Autodesk Fusion 360 part; units mm, degrees
(part 2 of 2)
  line L143 (-32.4194, -45.1753, 132.2927) -> (-24.3664, -49.1663, 133.2373) construction
  line L144 (-24.3664, -49.1663, 133.2373) -> (-16.3142, -53.1569, 134.1819) construction
  line L145 (-16.3142, -53.1569, 134.1819) -> (-7.27, -55.1267, 135.1265) construction
  line L146 (-7.27, -55.1267, 135.1265) -> (1.7125, -54.8463, 136.071) construction
  line L147 (1.7125, -54.8463, 136.071) -> (10.6942, -54.5658, 137.0155) construction
  line L148 (10.6942, -54.5658, 137.0155) -> (19.597, -52.0361, 137.96) construction
  line L149 (19.597, -52.0361, 137.96) -> (27.3842, -47.5516, 138.9044) construction
  line L150 (27.3842, -47.5516, 138.9044) -> (35.1706, -43.0675, 139.8488) construction
  line L151 (35.1706, -43.0675, 139.8488) -> (41.8265, -36.6377, 140.7932) construction
  line L152 (41.8265, -36.6377, 140.7932) -> (46.577, -29.0109, 141.7376) construction
  line L153 (46.577, -29.0109, 141.7376) -> (51.327, -21.3848, 142.6819) construction
  line L154 (51.327, -21.3848, 142.6819) -> (54.1627, -12.5764, 143.6262) construction
  line L155 (54.1627, -12.5764, 143.6262) -> (54.754, -3.6114, 144.5705) construction
  line L156 (54.754, -3.6114, 144.5705) -> (55.3453, 5.3528, 145.5148) construction
  line L157 (55.3453, 5.3528, 145.5148) -> (53.6914, 14.4564, 146.459) construction
  line L158 (53.6914, 14.4564, 146.459) -> (49.9848, 22.6398, 147.4032) construction
  line L159 (49.9848, 22.6398, 147.4032) -> (46.2786, 30.8225, 148.3474) construction
  line L160 (46.2786, 30.8225, 148.3474) -> (40.5272, 38.0694, 149.2915) construction
  line L161 (40.5272, 38.0694, 149.2915) -> (33.4001, 43.5371, 150.2356) construction
  line L162 (33.4001, 43.5371, 150.2356) -> (26.2735, 49.0044, 151.1797) construction
  line L163 (26.2735, 49.0044, 151.1797) -> (17.7851, 52.6822, 152.1238) construction
  line L164 (17.7851, 52.6822, 152.1238) -> (8.9225, 54.1427, 153.0678) construction
  line L165 (8.9225, 54.1427, 153.0678) -> (0.0607, 55.6031, 154.0118) construction
  line L166 (0.0607, 55.6031, 154.0118) -> (-9.1583, 54.8438, 154.9558) construction
  line L167 (-9.1583, 54.8438, 154.9558) -> (-17.6617, 51.953, 155.8998) construction
  line L168 (-17.6617, 51.953, 155.8998) -> (-26.1644, 49.0624, 156.8437) construction
  line L169 (-26.1644, 49.0624, 156.8437) -> (-33.9354, 44.0464, 157.7876) construction
  line L170 (-33.9354, 44.0464, 157.7876) -> (-40.0708, 37.4884, 158.7315) construction
  line L171 (-40.0708, 37.4884, 158.7315) -> (-46.2057, 30.9309, 159.6753) construction
  line L172 (-46.2057, 30.9309, 159.6753) -> (-50.6934, 22.8442, 160.6191) construction
  line L173 (-50.6934, 22.8442, 160.6191) -> (-53.0121, 14.1689, 161.5629) construction
  line L174 (-53.0121, 14.1689, 161.5629) -> (-55.3307, 5.4944, 162.5067) construction
  line L175 (-55.3307, 5.4944, 162.5067) -> (-55.476, -3.7522, 163.4504) construction
  line L176 (-55.476, -3.7522, 163.4504) -> (-53.4314, -12.4953, 164.3941) construction
  line L177 (-53.4314, -12.4953, 164.3941) -> (-51.3869, -21.2378, 165.3378) construction
  line L178 (-51.3869, -21.2378, 165.3378) -> (-47.1566, -29.4603, 166.2815) construction
  line L179 (-47.1566, -29.4603, 166.2815) -> (-41.2325, -36.2067, 167.2251) construction
  line L180 (-41.2325, -36.2067, 167.2251) -> (-35.3088, -42.9527, 168.1687) construction
  line L181 (-35.3088, -42.9527, 168.1687) -> (-27.7029, -48.2099, 169.1123) construction
  line L182 (-27.7029, -48.2099, 169.1123) -> (-19.2988, -51.3673, 170.0559) construction
  line L183 (-19.2988, -51.3673, 170.0559) -> (-10.8954, -54.5245, 170.9994) construction
  line L184 (-10.8954, -54.5245, 170.9994) -> (-1.7102, -55.5761, 171.9429) construction
  line L185 (-1.7102, -55.5761, 171.9429) -> (7.1893, -54.4, 172.8864) construction
  line L186 (7.1893, -54.4, 172.8864) -> (16.088, -53.224, 173.8298) construction
  line L187 (16.088, -53.224, 173.8298) -> (24.6841, -49.8228, 174.7733) construction
  line L188 (24.6841, -49.8228, 174.7733) -> (31.9784, -44.5918, 175.7167) construction
  line L189 (31.9784, -44.5918, 175.7167) -> (39.2722, -39.3611, 176.6601) construction
  line L190 (39.2722, -39.3611, 176.6601) -> (45.2505, -32.3109, 177.6034) construction
  line L191 (45.2505, -32.3109, 177.6034) -> (49.2187, -24.2604, 178.5468) construction
  line L192 (49.2187, -24.2604, 178.5468) -> (53.1866, -16.2104, 179.4901) construction
  line L193 (53.1866, -16.2104, 179.4901) -> (55.1371, -7.1757, 180.4333) construction
  line L194 (55.1371, -7.1757, 180.4333) -> (54.8437, 1.7942, 181.3766) construction
  line L195 (54.8437, 1.7942, 181.3766) -> (54.5502, 10.7635, 182.3198) construction
  line L196 (54.5502, 10.7635, 182.3198) -> (52.0137, 19.6507, 183.263) construction
  line L197 (52.0137, 19.6507, 183.263) -> (47.5288, 27.4237, 184.2062) construction
  line L198 (47.5288, 27.4237, 184.2062) -> (43.0443, 35.196, 185.1494) construction
  line L199 (43.0443, 35.196, 185.1494) -> (36.6202, 41.8393, 186.0925) construction
  line L200 (36.6202, 41.8393, 186.0925) -> (29.0026, 46.5821, 187.0356) construction
  line L201 (29.0026, 46.5821, 187.0356) -> (21.3857, 51.3245, 187.9787) construction
  line L202 (21.3857, 51.3245, 187.9787) -> (12.5901, 54.1576, 188.9218) construction
  line L203 (12.5901, 54.1576, 188.9218) -> (3.6372, 54.7523, 189.8648) construction
  line L204 (3.6372, 54.7523, 189.8648) -> (-5.315, 55.347, 190.8078) construction
  line L205 (-5.315, 55.347, 190.8078) -> (-14.4074, 53.7026, 191.7508) construction
  line L206 (-14.4074, 53.7026, 191.7508) -> (-22.5842, 50.01, 192.6938) construction
  line L207 (-22.5842, 50.01, 192.6938) -> (-30.7604, 46.3177, 193.6367) construction
  line L208 (-30.7604, 46.3177, 193.6367) -> (-38.0056, 40.5845, 194.5796) construction
  line L209 (-38.0056, 40.5845, 194.5796) -> (-43.4787, 33.4761, 195.5226) construction
  line L210 (-43.4787, 33.4761, 195.5226) -> (-48.9513, 26.3682, 196.4654) construction
  line L211 (-48.9513, 26.3682, 196.4654) -> (-52.6417, 17.8989, 197.4083) construction
  line L212 (-52.6417, 17.8989, 197.4083) -> (-54.1214, 9.0512, 198.3511) construction
  line L213 (-54.1214, 9.0512, 198.3511) -> (-55.6009, 0.2041, 199.2939) construction
  line L214 (-55.6009, 0.2041, 199.2939) -> (-54.8673, -9.0044, 200.2367) construction
  line L215 (-54.8673, -9.0044, 200.2367) -> (-52.0057, -17.5057, 201.1795) construction
  line L216 (-52.0057, -17.5057, 201.1795) -> (-49.1443, -26.0063, 202.1222) construction
  line L217 (-49.1443, -26.0063, 202.1222) -> (-44.1607, -33.7835, 203.0649) construction
  line L218 (-44.1607, -33.7835, 203.0649) -> (-37.6331, -39.9349, 204.0076) construction
  line L219 (-37.6331, -39.9349, 204.0076) -> (-31.106, -46.0858, 204.9502) construction
  line L220 (-31.106, -46.0858, 204.9502) -> (-23.0477, -50.5993, 205.8929) construction
  line L221 (-23.0477, -50.5993, 205.8929) -> (-14.3931, -52.9517, 206.8355) construction
  line L222 (-14.3931, -52.9517, 206.8355) -> (-5.7391, -55.304, 207.7781) construction
  line L223 (-5.7391, -55.304, 207.7781) -> (3.4946, -55.4911, 208.7207) construction
  line L224 (3.4946, -55.4911, 208.7207) -> (12.2368, -53.4912, 209.6632) construction
  line L225 (12.2368, -53.4912, 209.6632) -> (20.9783, -51.4915, 210.6058) construction
  line L226 (20.9783, -51.4915, 210.6058) -> (29.2118, -47.3089, 211.5483) construction
  line L227 (29.2118, -47.3089, 211.5483) -> (35.9821, -41.4287, 212.4908) construction
  line L228 (35.9821, -41.4287, 212.4908) -> (42.7519, -35.5489, 213.4332) construction
  line L229 (42.7519, -35.5489, 213.4332) -> (48.0459, -27.9829, 214.3757) construction
  line L230 (48.0459, -27.9829, 214.3757) -> (51.25, -19.6082, 215.3181) construction
  line L231 (51.25, -19.6082, 215.3181) -> (54.4539, -11.2341, 216.2605) construction
  line L232 (54.4539, -11.2341, 216.2605) -> (55.5622, -2.0673, 217.2029) construction
  line L233 (55.5622, -2.0673, 217.2029) -> (54.4464, 6.8291, 218.1452) construction
  line L234 (54.4464, 6.8291, 218.1452) -> (53.3306, 15.7249, 219.0875) construction
  line L235 (53.3306, 15.7249, 219.0875) -> (49.9931, 24.3334, 220.0299) construction
  line L236 (49.9931, 24.3334, 220.0299) -> (44.8209, 31.6565, 220.9722) construction
  line L237 (44.8209, 31.6565, 220.9722) -> (39.649, 38.9791, 221.9144) construction
  line L238 (39.649, 38.9791, 221.9144) -> (32.6524, 45.0026, 222.8567) construction
  line L239 (32.6524, 45.0026, 222.8567) -> (24.6424, 49.0285, 223.7989) construction
  line L240 (24.6424, 49.0285, 223.7989) -> (16.6329, 53.0542, 224.7411) construction
  line L241 (16.6329, 53.0542, 224.7411) -> (7.6252, 55.075, 225.6833) construction
  line L242 (7.6252, 55.075, 225.6833) -> (-1.3364, 54.8567, 226.6255) construction
  line L243 (-1.3364, 54.8567, 226.6255) -> (-10.2974, 54.6384, 227.5676) construction
  line L244 (-10.2974, 54.6384, 227.5676) -> (-19.1954, 52.1817, 228.5097) construction
  line L245 (-19.1954, 52.1817, 228.5097) -> (-26.999, 47.7713, 229.4518) construction
  line L246 (-26.999, 47.7713, 229.4518) -> (-34.8021, 43.3612, 230.3939) construction
  line L247 (-34.8021, 43.3612, 230.3939) -> (-41.4962, 37.0061, 231.336) construction
  line L248 (-41.4962, 37.0061, 231.336) -> (-46.3054, 29.4425, 232.278) construction
  line L249 (-46.3054, 29.4425, 232.278) -> (-51.1143, 21.8793, 233.22) construction
  line L250 (-51.1143, 21.8793, 233.22) -> (-54.0294, 13.1222, 234.162) construction
  line L251 (-54.0294, 13.1222, 234.162) -> (-54.7131, 4.1858, 235.104) construction
  line L252 (-54.7131, 4.1858, 235.104) -> (-55.3967, -4.7501, 236.046) construction
  line L253 (-55.3967, -4.7501, 236.046) -> (-53.8479, -13.8482, 236.9879) construction
  line L254 (-53.8479, -13.8482, 236.9879) -> (-50.2459, -22.0544, 237.9298) construction
  line L255 (-50.2459, -22.0544, 237.9298) -> (-46.6442, -30.2601, 238.8717) construction
  line L256 (-46.6442, -30.2601, 238.8717) -> (-40.9965, -37.5585, 239.8136) construction
  line L257 (-40.9965, -37.5585, 239.8136) -> (-33.9571, -43.1041, 240.7555) construction
  line L258 (-33.9571, -43.1041, 240.7555) -> (-26.9181, -48.6493, 241.6973) construction
  line L259 (-26.9181, -48.6493, 241.6973) -> (-18.501, -52.4314, 242.6391) construction
  line L260 (-18.501, -52.4314, 242.6391) -> (-9.6808, -54.0123, 243.581) construction
  line L261 (-9.6808, -54.0123, 243.581) -> (-0.8611, -55.5931, 244.5227) construction
  line L262 (-0.8611, -55.5931, 244.5227) -> (8.345, -54.9699, 245.4645) construction
  line L263 (8.345, -54.9699, 245.4645) -> (16.8713, -52.215, 246.4062) construction
  line L264 (16.8713, -52.215, 246.4062) -> (25.397, -49.4602, 247.3479) construction
  line L265 (25.397, -49.4602, 247.3479) -> (33.2267, -44.5792, 248.2897) construction
  line L266 (33.2267, -44.5792, 248.2897) -> (39.4538, -38.1372, 249.2314) construction
  line L267 (39.4538, -38.1372, 249.2314) -> (45.6805, -31.6955, 250.173) construction
  line L268 (45.6805, -31.6955, 250.173) -> (50.2929, -23.7052, 251.1147) construction
  line L269 (50.2929, -23.7052, 251.1147) -> (52.7569, -15.0915, 252.0563) construction
  line L270 (52.7569, -15.0915, 252.0563) -> (55.2208, -6.4784, 252.9979) construction
  line L271 (55.2208, -6.4784, 252.9979) -> (55.5318, 2.7418, 253.9395) construction
  line L272 (55.5318, 2.7418, 253.9395) -> (53.6541, 11.5014, 254.8811) construction
  line L273 (53.6541, 11.5014, 254.8811) -> (51.7765, 20.2606, 255.8226) construction
  line L274 (51.7765, 20.2606, 255.8226) -> (47.7139, 28.5426, 256.7642) construction
  line L275 (47.7139, 28.5426, 256.7642) -> (41.9366, 35.3888, 257.7057) construction
  line L276 (41.9366, 35.3888, 257.7057) -> (36.1596, 42.2347, 258.6472) construction
  line L277 (36.1596, 42.2347, 258.6472) -> (28.6791, 47.6318, 259.5887) construction
  line L278 (28.6791, 47.6318, 259.5887) -> (20.361, 50.9556, 260.5301) construction
  line L279 (20.361, 50.9556, 260.5301) -> (12.0434, 54.2792, 261.4716) construction
  line L280 (12.0434, 54.2792, 261.4716) -> (2.904, 55.5233, 262.413) construction
  line L281 (2.904, 55.5233, 262.413) -> (-5.9994, 54.5441, 263.3544) construction
  line L282 (-5.9994, 54.5441, 263.3544) -> (-14.9023, 53.5648, 264.2958) construction
  line L283 (-14.9023, 53.5648, 264.2958) -> (-23.5523, 50.3642, 265.2372) construction
  line L284 (-23.5523, 50.3642, 265.2372) -> (-30.9484, 45.3127, 266.1785) construction
  line L285 (-30.9484, 45.3127, 266.1785) -> (-38.3441, 40.2615, 267.1199) construction
  line L286 (-38.3441, 40.2615, 267.1199) -> (-44.472, 33.3691, 268.0612) construction
  line L287 (-44.472, 33.3691, 268.0612) -> (-48.6231, 25.4331, 269.0025) construction
  line L288 (-48.6231, 25.4331, 269.0025) -> (-52.7739, 17.4976, 269.9438) construction
  line L289 (-52.7739, 17.4976, 269.9438) -> (-54.9402, 8.5336, 270.8851) construction
  line L290 (-54.9402, 8.5336, 270.8851) -> (-54.8714, -0.4217, 271.8263) construction
  line L291 (-54.8714, -0.4217, 271.8263) -> (-54.8026, -9.3765, 272.7675) construction
  line L292 (-54.8026, -9.3765, 272.7675) -> (-52.499, -18.3057, 273.7088) construction
  line L293 (-52.499, -18.3057, 273.7088) -> (-48.2271, -26.1762, 274.65) construction
  line L294 (-48.2271, -26.1762, 274.65) -> (-43.9555, -34.0463, 275.5911) construction
  line L295 (-43.9555, -34.0463, 275.5911) -> (-37.7238, -40.8429, 276.5323) construction
  line L296 (-37.7238, -40.8429, 276.5323) -> (-30.2531, -45.7798, 277.4735) construction
  line L297 (-30.2531, -45.7798, 277.4735) -> (-22.7828, -50.7165, 278.4146) construction
  line L298 (-22.7828, -50.7165, 278.4146) -> (-14.0877, -53.7844, 279.3557) construction
  line L299 (-14.0877, -53.7844, 279.3557) -> (-5.1734, -54.6286, 280.2968) construction
  line L300 (-5.1734, -54.6286, 280.2968) -> (3.7404, -55.4727, 281.2379) construction
  line L301 (3.7404, -55.4727, 281.2379) -> (12.8563, -54.0919, 282.179) construction
  line L302 (12.8563, -54.0919, 282.179) -> (21.1202, -50.6457, 283.12) construction
  line L303 (21.1202, -50.6457, 283.12) -> (29.3837, -47.1996, 284.0611) construction
  line L304 (29.3837, -47.1996, 284.0611) -> (36.7795, -41.695, 285.0021) construction
  line L305 (36.7795, -41.695, 285.0021) -> (42.4524, -34.7684, 285.9431) construction
  line L306 (42.4524, -34.7684, 285.9431) -> (48.125, -27.8421, 286.8841) construction
  line L307 (48.125, -27.8421, 286.8841) -> (52.0641, -19.5071, 287.8251) construction
  line L308 (52.0641, -19.5071, 287.8251) -> (53.8143, -10.7271, 288.766) construction
  line L309 (53.8143, -10.7271, 288.766) -> (55.5644, -1.9475, 289.707) construction
  line L310 (55.5644, -1.9475, 289.707) -> (55.1224, 7.2604, 290.6479) construction
  line L311 (55.1224, 7.2604, 290.6479) -> (52.5395, 15.832, 291.5888) construction
  line L312 (52.5395, 15.832, 291.5888) -> (49.8436, 24.7785, 292.5709) construction
  line L313 (49.8436, 24.7785, 292.5709) -> (44.8171, 33.0118, 293.553) construction
  line L314 (44.8171, 33.0118, 293.553) -> (38.0914, 39.498, 294.535) construction
  line L315 (38.0914, 39.498, 294.535) -> (31.4707, 45.8829, 295.5018) construction
  line L316 (31.4707, 45.8829, 295.5018) -> (23.2186, 50.5623, 296.4685) construction
  line L317 (23.2186, 50.5623, 296.4685) -> (14.3404, 52.966, 297.4353) construction
  line L318 (14.3404, 52.966, 297.4353) -> (5.6009, 55.3322, 298.3869) construction
  line L319 (5.6009, 55.3322, 298.3869) -> (-3.7272, 55.4899, 299.3385) construction
  line L320 (-3.7272, 55.4899, 299.3385) -> (-12.5417, 53.4205, 300.2901) construction
  line L321 (-12.5417, 53.4205, 300.2901) -> (-21.2944, 51.3656, 301.2351) construction
  line L322 (-21.2944, 51.3656, 301.2351) -> (-29.5237, 47.1193, 302.1801) construction
  line L323 (-29.5237, 47.1193, 302.1801) -> (-36.2702, 41.1766, 303.125) construction
  line L324 (-36.2702, 41.1766, 303.125) -> (-43.0156, 35.2351, 304.0698) construction
  line L325 (-43.0156, 35.2351, 304.0698) -> (-48.2657, 27.6092, 305.0146) construction
  line L326 (-48.2657, 27.6092, 305.0146) -> (-51.4089, 19.1877, 305.9594) construction
  line L327 (-51.4089, 19.1877, 305.9594) -> (-54.5516, 10.7677, 306.904) construction
  line L328 (-54.5516, 10.7677, 306.904) -> (-55.582, 1.5686, 307.8486) construction
  line L329 (-55.582, 1.5686, 307.8486) -> (-54.3801, -7.338, 308.7932) construction
  line L330 (-54.3801, -7.338, 308.7932) -> (-53.1785, -16.243, 309.7376) construction
  line L331 (-53.1785, -16.243, 309.7376) -> (-49.7478, -24.8384, 310.682) construction
  line L332 (-49.7478, -24.8384, 310.682) -> (-44.4874, -32.1234, 311.6265) construction
  line L333 (-44.4874, -32.1234, 311.6265) -> (-39.228, -39.4072, 312.5707) construction
  line L334 (-39.228, -39.4072, 312.5707) -> (-32.1497, -45.3669, 313.515) construction
  line L335 (-32.1497, -45.3669, 313.515) -> (-24.0766, -49.3088, 314.4593) construction
  line L336 (-24.0766, -49.3088, 314.4593) -> (-16.005, -53.2501, 315.4034) construction
  line L337 (-16.005, -53.2501, 315.4034) -> (-6.9543, -55.1667, 316.3475) construction
  line L338 (-6.9543, -55.1667, 316.3475) -> (2.0222, -54.8357, 317.2916) construction
  line L339 (2.0222, -54.8357, 317.2916) -> (10.997, -54.5048, 318.2355) construction
  line L340 (10.997, -54.5048, 318.2355) -> (19.8805, -51.9276, 319.1795) construction
  line L341 (19.8805, -51.9276, 319.1795) -> (27.639, -47.4039, 320.1234) construction
  line L342 (27.639, -47.4039, 320.1234) -> (35.3962, -42.8811, 321.0672) construction
  line L343 (35.3962, -42.8811, 321.0672) -> (42.0141, -36.4211, 322.011) construction
  line L344 (42.0141, -36.4211, 322.011) -> (46.7229, -28.7753, 322.9548) construction
  line L345 (46.7229, -28.7753, 322.9548) -> (51.4309, -21.1308, 323.8984) construction
  line L346 (51.4309, -21.1308, 323.8984) -> (54.2216, -12.3155, 324.842) construction
  line L347 (54.2216, -12.3155, 324.842) -> (54.7704, -3.3543, 325.7856) construction
  line L348 (54.7704, -3.3543, 325.7856) -> (55.3191, 5.6054, 326.7291) construction
  line L349 (55.3191, 5.6054, 326.7291) -> (53.6257, 14.6938, 327.6726) construction
  line L350 (53.6257, 14.6938, 327.6726) -> (49.887, 22.8547, 328.616) construction
  line L351 (49.887, 22.8547, 328.616) -> (46.1488, 31.0143, 329.5594) construction
  line L352 (46.1488, 31.0143, 329.5594) -> (40.3732, 38.2309, 330.5027) construction
  line L353 (40.3732, 38.2309, 330.5027) -> (33.2311, 43.6663, 331.446) construction
  line L354 (33.2311, 43.6663, 331.446) -> (26.0901, 49.1007, 332.3892) construction
  line L355 (26.0901, 49.1007, 332.3892) -> (17.5967, 52.744, 333.3323) construction
  line L356 (17.5967, 52.744, 333.3323) -> (8.7376, 54.1729, 334.2755) construction
  line L357 (8.7376, 54.1729, 334.2755) -> (-0.1203, 55.6016, 335.2185) construction
  line L358 (-0.1203, 55.6016, 335.2185) -> (-9.3269, 54.8138, 336.1616) construction
  line L359 (-9.3269, 54.8138, 336.1616) -> (-17.8133, 51.9012, 337.1046) construction
  line L360 (-17.8133, 51.9012, 337.1046) -> (-26.2984, 48.989, 338.0475) construction
  line L361 (-26.2984, 48.989, 338.0475) -> (-34.0472, 43.958, 338.9904) construction
  line L362 (-34.0472, 43.958, 338.9904) -> (-40.1604, 37.3924, 339.9333) construction
  line L363 (-40.1604, 37.3924, 339.9333) -> (-46.2726, 30.8277, 340.876) construction
  line L364 (-46.2726, 30.8277, 340.876) -> (-50.7379, 22.7413, 341.8188) construction
  line L365 (-50.7379, 22.7413, 341.8188) -> (-53.0381, 14.0716, 342.7615) construction
  line L366 (-53.0381, 14.0716, 342.7615) -> (-55.3379, 5.4032, 343.7041) construction
  line L367 (-55.3379, 5.4032, 343.7041) -> (-55.4689, -3.8318, 344.6467) construction
  line L368 (-55.4689, -3.8318, 344.6467) -> (-53.4158, -12.562, 345.5893) construction
  line L369 (-53.4158, -12.562, 345.5893) -> (-51.3629, -21.2909, 346.5318) construction
  line L370 (-51.3629, -21.2909, 346.5318) -> (-47.1306, -29.4985, 347.4743) construction
  line L371 (-47.1306, -29.4985, 347.4743) -> (-41.2097, -36.2327, 348.4168) construction
  line L372 (-41.2097, -36.2327, 348.4168) -> (-35.2895, -42.9661, 349.3591) construction
  line L373 (-35.2895, -42.9661, 349.3591) -> (-27.6925, -48.2137, 350.3015) construction
  line L374 (-27.6925, -48.2137, 350.3015) -> (-19.2995, -51.3671, 351.2438) construction
  line L375 (-19.2995, -51.3671, 351.2438) -> (-10.9077, -54.52, 352.186) construction
  line L376 (-10.9077, -54.52, 352.186) -> (-1.7361, -55.5733, 353.1282) construction
  line L377 (-1.7361, -55.5733, 353.1282) -> (7.152, -54.4049, 354.0705) construction
  line L378 (7.152, -54.4049, 354.0705) -> (16.039, -53.2366, 355.0125) construction
  line L379 (16.039, -53.2366, 355.0125) -> (24.6256, -49.8494, 355.9546) construction
  line L380 (24.6256, -49.8494, 355.9546) -> (31.9168, -44.6359, 356.8967) construction
  line L381 (31.9168, -44.6359, 356.8967) -> (39.2071, -39.423, 357.8387) construction
  line L382 (39.2071, -39.423, 357.8387) -> (45.1883, -32.3942, 358.7807) construction
  line L383 (45.1883, -32.3942, 358.7807) -> (49.1676, -24.3638, 359.7226) construction
  line L384 (49.1676, -24.3638, 359.7226) -> (53.1464, -16.3344, 360.6645) construction
  line L385 (53.1464, -16.3344, 360.6645) -> (55.1161, -7.319, 361.6064) construction
  line L386 (55.1161, -7.319, 361.6064) -> (54.8485, 1.6381, 362.5482) construction
  line L387 (54.8485, 1.6381, 362.5482) -> (54.5811, 10.5941, 363.4899) construction
  line L388 (54.5811, 10.5941, 363.4899) -> (52.0774, 19.4749, 364.4317) construction
  line L389 (52.0774, 19.4749, 364.4317) -> (47.6276, 27.2518, 365.3734) construction
  line L390 (47.6276, 27.2518, 365.3734) -> (43.1783, 35.0278, 366.315) construction
  line L391 (43.1783, 35.0278, 366.315) -> (36.7917, 41.6855, 367.2566) construction
  line L392 (36.7917, 41.6855, 367.2566) -> (29.2073, 46.454, 368.1983) construction
  line L393 (29.2073, 46.454, 368.1983) -> (21.6238, 51.2221, 369.1398) construction
  line L394 (21.6238, 51.2221, 369.1398) -> (12.8572, 54.0923, 370.0813) construction
  line L395 (12.8572, 54.0923, 370.0813) -> (3.9223, 54.7326, 371.0228) construction
  line L396 (3.9223, 54.7326, 371.0228) -> (-5.0117, 55.3729, 371.9642) construction
  line L397 (-5.0117, 55.3729, 371.9642) -> (-14.0969, 53.7824, 372.9056) construction
  line L398 (-14.0969, 53.7824, 372.9056) -> (-22.2821, 50.1453, 373.847) construction
  line L399 (-22.2821, 50.1453, 373.847) -> (-30.4663, 46.5087, 374.7883) construction
  line L400 (-30.4663, 46.5087, 374.7883) -> (-37.7351, 40.8328, 375.7296) construction
  line L401 (-37.7351, 40.8328, 375.7296) -> (-43.2474, 33.7744, 376.6709) construction
  line L402 (-43.2474, 33.7744, 376.6709) -> (-48.7591, 26.7167, 377.6121) construction
  line L403 (-48.7591, 26.7167, 377.6121) -> (-52.5043, 18.2902, 378.5533) construction
  line L404 (-52.5043, 18.2902, 378.5533) -> (-54.0497, 9.4697, 379.4945) construction
  line L405 (-54.0497, 9.4697, 379.4945) -> (-55.5949, 0.6502, 380.4356) construction
  line L406 (-55.5949, 0.6502, 380.4356) -> (-54.9379, -8.5466, 381.3767) construction
  line L407 (-54.9379, -8.5466, 381.3767) -> (-52.1546, -17.057, 382.3178) construction
  line L408 (-52.1546, -17.057, 382.3178) -> (-49.3717, -25.5664, 383.2588) construction
  line L409 (-49.3717, -25.5664, 383.2588) -> (-44.4681, -33.3735, 384.1998) construction
  line L410 (-44.4681, -33.3735, 384.1998) -> (-38.0111, -39.5753, 385.1408) construction
  line L411 (-38.0111, -39.5753, 385.1408) -> (-31.2201, -46.0978, 386.1304) construction
  line L412 (-31.2201, -46.0978, 386.1304) -> (-22.7221, -50.8273, 387.1201) construction
  line L413 (-22.7221, -50.8273, 387.1201) -> (-13.5999, -53.161, 388.1097) construction
  line L414 (-13.5999, -53.161, 388.1097) -> (-4.7627, -55.4217, 389.0685) construction
  line L415 (-4.7627, -55.4217, 389.0685) -> (4.6405, -55.4321, 390.0272) construction
  line L416 (4.6405, -55.4321, 390.0272) -> (13.4826, -53.1908, 390.9859) construction
  line L417 (13.4826, -53.1908, 390.9859) -> (22.1968, -50.982, 391.9308) construction
  line L418 (22.1968, -50.982, 391.9308) -> (30.3491, -46.5918, 392.8757) construction
  line L419 (30.3491, -46.5918, 392.8757) -> (36.9893, -40.5319, 393.8205) construction
  line L420 (36.9893, -40.5319, 393.8205) -> (43.6272, -34.4742, 394.765) construction
  line L421 (43.6272, -34.4742, 394.765) -> (48.7413, -26.7598, 395.7096) construction
  line L422 (48.7413, -26.7598, 395.7096) -> (51.7361, -18.2871, 396.6541) construction
  line L423 (51.7361, -18.2871, 396.6541) -> (54.7299, -9.8174, 397.5982) construction
  line L424 (54.7299, -9.8174, 397.5982) -> (55.6002, -0.6062, 398.5424) construction
  line L425 (55.6002, -0.6062, 398.5424) -> (54.2456, 8.2743, 399.4866) construction
  line L426 (54.2456, 8.2743, 399.4866) -> (52.8914, 17.1518, 400.4305) construction
  line L427 (52.8914, 17.1518, 400.4305) -> (49.3167, 25.6818, 401.3743) construction
  line L428 (49.3167, 25.6818, 401.3743) -> (43.937, 32.8723, 402.3182) construction
  line L429 (43.937, 32.8723, 402.3182) -> (38.5591, 40.0603, 403.2617) construction
  line L430 (38.5591, 40.0603, 403.2617) -> (31.3879, 45.8959, 404.2052) construction
  line L431 (31.3879, 45.8959, 404.2052) -> (23.2569, 49.7007, 405.1488) construction
  line L432 (23.2569, 49.7007, 405.1488) -> (15.1285, 53.5043, 406.092) construction
  line L433 (15.1285, 53.5043, 406.092) -> (6.0564, 55.2712, 407.0353) construction
  line L434 (6.0564, 55.2712, 407.0353) -> (-2.9053, 54.796, 407.9785) construction
  line L435 (-2.9053, 54.796, 407.9785) -> (-11.8643, 54.321, 408.9215) construction
  line L436 (-11.8643, 54.321, 408.9215) -> (-20.6959, 51.6063, 409.8644) construction
  line L437 (-20.6959, 51.6063, 409.8644) -> (-28.3749, 46.9671, 410.8074) construction
  line L438 (-28.3749, 46.9671, 410.8074) -> (-36.0516, 42.3293, 411.75) construction
  line L439 (-36.0516, 42.3293, 411.75) -> (-42.5617, 35.7769, 412.6927) construction
  line L440 (-42.5617, 35.7769, 412.6927) -> (-47.1498, 28.0704, 413.6354) construction
  line L441 (-47.1498, 28.0704, 413.6354) -> (-51.7365, 20.366, 414.5778) construction
  line L442 (-51.7365, 20.366, 414.5778) -> (-54.3936, 11.5227, 415.5202) construction
  line L443 (-54.3936, 11.5227, 415.5202) -> (-54.813, 2.5661, 416.4626) construction
  line L444 (-54.813, 2.5661, 416.4626) -> (-55.2322, -6.388, 417.4047) construction
  line L445 (-55.2322, -6.388, 417.4047) -> (-53.414, -15.4383, 418.3469) construction
  line L446 (-53.414, -15.4383, 418.3469) -> (-49.5692, -23.5359, 419.289) construction
  line L447 (-49.5692, -23.5359, 419.289) -> (-45.7255, -31.6313, 420.2309) construction
  line L448 (-45.7255, -31.6313, 420.2309) -> (-39.8634, -38.759, 421.1729) construction
  line L449 (-39.8634, -38.759, 421.1729) -> (-32.6623, -44.0933, 422.1148) construction
  line L450 (-32.6623, -44.0933, 422.1148) -> (-25.4629, -49.4263, 423.0564) construction
  line L451 (-25.4629, -49.4263, 423.0564) -> (-16.9388, -52.9565, 423.9981) construction
  line L452 (-16.9388, -52.9565, 423.9981) -> (-8.077, -54.2753, 424.9398) construction
  line L453 (-8.077, -54.2753, 424.9398) -> (0.7827, -55.5938, 425.8812) construction
  line L454 (0.7827, -55.5938, 425.8812) -> (9.9632, -54.6993, 426.8227) construction
  line L455 (9.9632, -54.6993, 426.8227) -> (18.4018, -51.6955, 427.7641) construction
  line L456 (18.4018, -51.6955, 427.7641) -> (26.8385, -48.6923, 428.7054) construction
  line L457 (26.8385, -48.6923, 428.7054) -> (34.5177, -43.5864, 429.6466) construction
  line L458 (34.5177, -43.5864, 429.6466) -> (40.551, -36.9684, 430.5879) construction
  line L459 (40.551, -36.9684, 430.5879) -> (46.583, -30.3519, 431.5289) construction
  line L460 (46.583, -30.3519, 431.5289) -> (50.9583, -22.2365, 432.4699) construction
  line L461 (50.9583, -22.2365, 432.4699) -> (53.171, -13.5608, 433.411) construction
  line L462 (53.171, -13.5608, 433.411) -> (55.4604, -4.5841, 434.3847) construction
  line L463 (55.4604, -4.5841, 434.3847) -> (55.4267, 4.9747, 435.3584) construction
  line L464 (55.4267, 4.9747, 435.3584) -> (53.0741, 13.935, 436.3321) construction
  line L465 (53.0741, 13.935, 436.3321) -> (50.7916, 22.6283, 437.2767) construction
  line L466 (50.7916, 22.6283, 437.2767) -> (46.3335, 30.7415, 438.2214) construction
  line L467 (46.3335, 30.7415, 438.2214) -> (40.2191, 37.3292, 439.1661) construction
  line L468 (40.2191, 37.3292, 439.1661) -> (34.1091, 43.9122, 440.1101) construction
  line L469 (34.1091, 43.9122, 440.1101) -> (26.357, 48.9594, 441.0541) construction
  line L470 (26.357, 48.9594, 441.0541) -> (17.8648, 51.8835, 441.9981) construction
  line L471 (17.8648, 51.8835, 441.9981) -> (9.3782, 54.8056, 442.9414) construction
  line L472 (9.3782, 54.8056, 442.9414) -> (0.1687, 55.602, 443.8848) construction
  line L473 (0.1687, 55.602, 443.8848) -> (-8.6936, 54.18, 444.8282) construction
  line L474 (-8.6936, 54.18, 444.8282) -> (-17.5504, 52.7588, 445.771) construction
  line L475 (-17.5504, 52.7588, 445.771) -> (-26.0435, 49.1248, 446.7138) construction
  line L476 (-26.0435, 49.1248, 446.7138) -> (-33.1871, 43.6997, 447.6566) construction
  line L477 (-33.1871, 43.6997, 447.6566) -> (-40.3267, 38.2776, 448.5989) construction
  line L478 (-40.3267, 38.2776, 448.5989) -> (-46.1047, 31.0768, 449.5411) construction
  line L479 (-46.1047, 31.0768, 449.5411) -> (-49.8514, 22.9322, 450.4834) construction
  line L480 (-49.8514, 22.9322, 450.4834) -> (-53.5961, 14.7918, 451.4252) construction
  line L481 (-53.5961, 14.7918, 451.4252) -> (-55.3043, 5.724, 452.367) construction
  line L482 (-55.3043, 5.724, 452.367) -> (-54.7784, -3.221, 453.3087) construction
  line L483 (-54.7784, -3.221, 453.3087) -> (-54.2527, -12.1617, 454.2501) construction
  line L484 (-54.2527, -12.1617, 454.2501) -> (-51.4958, -20.9628, 455.1914) construction
  line L485 (-51.4958, -20.9628, 455.1914) -> (-46.8269, -28.6057, 456.1327) construction
  line L486 (-46.8269, -28.6057, 456.1327) -> (-42.1599, -36.2454, 457.0737) construction
  line L487 (-42.1599, -36.2454, 457.0737) -> (-35.5913, -42.7136, 458.0146) construction
  line L488 (-35.5913, -42.7136, 458.0146) -> (-27.8806, -47.2622, 458.9556) construction
  line L489 (-27.8806, -47.2622, 458.9556) -> (-20.1421, -51.8273, 459.8999) construction
  line L490 (-20.1421, -51.8273, 459.8999) -> (-11.2678, -54.45, 460.8442) construction
  line L491 (-11.2678, -54.45, 460.8442) -> (-2.291, -54.8252, 461.7885) construction
  line L492 (-2.291, -54.8252, 461.7885) -> (6.674, -55.1998, 462.7316) construction
  line L493 (6.674, -55.1998, 462.7316) -> (15.7241, -53.3321, 463.6747) construction
  line L494 (15.7241, -53.3321, 463.6747) -> (23.8083, -49.439, 464.6178) construction
  line L495 (23.8083, -49.439, 464.6178) -> (31.8834, -45.5503, 465.5598) construction
  line L496 (31.8834, -45.5503, 465.5598) -> (38.9794, -39.6482, 466.5018) construction
  line L497 (38.9794, -39.6482, 466.5018) -> (44.2742, -32.4167, 467.4438) construction
  line L498 (44.2742, -32.4167, 467.4438) -> (49.564, -25.192, 468.3849) construction
  line L499 (49.564, -25.192, 468.3849) -> (53.0459, -16.6541, 469.3261) construction
  line L500 (53.0459, -16.6541, 469.3261) -> (54.3172, -7.7906, 470.2672) construction
  line L501 (54.3172, -7.7906, 470.2672) -> (55.5919, 1.0969, 471.2109) construction
  line L502 (55.5919, 1.0969, 471.2109) -> (54.6413, 10.2949, 472.1546) construction
  line L503 (54.6413, 10.2949, 472.1546) -> (51.576, 18.7339, 473.0982) construction
  line L504 (51.576, 18.7339, 473.0982) -> (48.5177, 27.1538, 474.0398) construction
  line L505 (48.5177, 27.1538, 474.0398) -> (43.3601, 34.8023, 474.9813) construction
  line L506 (43.3601, 34.8023, 474.9813) -> (36.7004, 40.7937, 475.9229) construction
  line L507 (36.7004, 40.7937, 475.9229) -> (30.0339, 46.7913, 476.8654) construction
  line L508 (30.0339, 46.7913, 476.8654) -> (21.8748, 51.117, 477.8079) construction
  line L509 (21.8748, 51.117, 477.8079) -> (13.1696, 53.2692, 478.7504) construction
  line L510 (13.1696, 53.2692, 478.7504) -> (8.866, 54.3332, 479.2163) construction
  line L511 (8.866, 54.3332, 479.2163) -> (4.4331, 54.873, 479.6823) construction
  line L512 (4.4331, 54.873, 479.6823) -> (0, 54.873, 480.1482) construction
  spline S1 degree 5 poles (51.2639, 19.5586, 2.1021) (51.7733, 18.2198, 1.9515) (52.6774, 15.6379, 1.4563) (53.6897, 12.0523, 0.1318) (54.4535, 7.8214, -2.6536) (54.8056, 3.5313, -7.3829) (54.8617, 1.1604, -11.9502) (54.8709, 0.2111, -15.8003) (54.873, 0, -18.5668) (54.873, 0, -20) knots 0 0 0 0 0 0 0.2 0.4 0.6 0.8 1 1 1 1 1 1
  dimension "d7" = 20
  dimension "d8" = 20
  dimension "d9" = 19.9996
delete_body "Körper entfernen1" bodies 1
pipe "Leitung1" add diameter 6 path "Skizze2" along L1 S1 S0 separate body makes body 2
named bodies: "Spiral Triangle", "Copper Wire"
